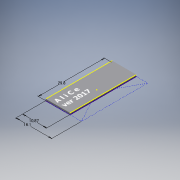
# Autodesk Inventor part: monitor
Saved by Autodesk Inventor 2016 (Build 200138000, 138)
## iProperties
Created: 2017-06-12
Part Number: monitor
Material: 一般
Document SubType Name: Modeling
Designer: B4_Ohno
Density: 1 g/cm^3
Appearance: 既定
Author: B4_Ohno
Autodesk Inventor part; units mm, degrees
ref_plane "YZ Plane" through (0, 0, 0) normal (1, 0, 0) x (0, 1, 0)
ref_plane "XZ Plane" through (0, 0, 0) normal (0, 1, 0) x (-1, 0, 0)
ref_plane "XY Plane" through (0, 0, 0) normal (0, 0, 1) x (1, 0, 0)
sketch "スケッチ1" plane through (0, 0, 0) normal (0, 0, 1) x (1, 0, 0)
  line L0 (8.05, 14.9) -> (-8.05, 14.9) construction
  line L1 (-8.05, 14.9) -> (-8.05, -14.9) construction
  line L2 (-8.05, -14.9) -> (8.05, -14.9) construction
  line L3 (8.05, -14.9) -> (8.05, 14.9) construction
  line L4 (8.05, 14.9) -> (-8.05, -14.9) construction
  line L5 (-8.05, 14.9) -> (8.05, -14.9) construction
  line L6 (2.82, 14.9) -> (-8.05, 14.9)
  line L7 (-8.05, 14.9) -> (-8.05, -14.9)
  line L8 (-8.05, -14.9) -> (2.82, -14.9)
  line L9 (2.82, -14.9) -> (2.82, 14.9)
  point P0 (0, 0)
  dimension "d0" = 16.1
  dimension "d1" = 29.8
  dimension "d2" = 10.87
  constraints: 20 end point, 4 parallel, 2 horizontal, 2 midpoint, 2 perpendicular
  measures "d0" distance of L2.end L1.end
  measures "d1" distance of L0.end L1.end
  measures "d2" distance of L1.end L8.end
extrude "押し出し1" add sketch "スケッチ1" along normal blind 0.725
sketch "スケッチ3" plane through (0, 0, 0.725) normal (0, 0, 1) x (1, 0, 0)
  line L0 (-5.93, -13.79) -> (-5.93, 13.79) construction
  line L1 (-5.93, 13.79) -> (0.7, 13.79) construction
  line L2 (0.7, 13.79) -> (0.7, -13.79) construction
  line L3 (0.7, -13.79) -> (-5.93, -13.79) construction
  line L4 (2.82, -14.9) -> (2.82, 14.9) projected
  line L5 (-8.05, 14.9) -> (-8.05, -14.9) projected
  point P0 (0, 0)
  dimension "d5" = 2.12
  dimension "d6" = 2.12
  dimension "d7" = 1.11
  dimension "d8" = 1.11
  constraints: 1 perpendicular, 2 other
  measures "d5" distance between parallel lines of L5 L0
  measures "d6" distance between parallel lines of L4 L2
  measures "d7" vertical distance of L5.end L0.start
  measures "d8" vertical distance of L5.start L0.end
equation "\"d6\" = d5"
equation "\"d8\" = d7"
